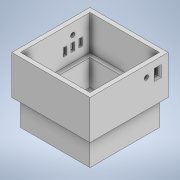
# Autodesk Inventor part: BlackBoxBottomFall2019
Saved by Autodesk Inventor 2020 (Build 240168000, 168)
## iProperties
Created: 2019-08-26
Part Number: BlackBoxBottomFall2019
Material: Generic
Document SubType Name: Modeling
Designer: hwatsky
Density: 1 g/cm^3
Appearance: Default
Author: hwatsky
Autodesk Inventor part; units mm, degrees
ref_plane "YZ Plane" through (0, 0, 0) normal (1, 0, 0) x (0, 1, 0)
ref_plane "XZ Plane" through (0, 0, 0) normal (0, 1, 0) x (-1, 0, 0)
ref_plane "XY Plane" through (0, 0, 0) normal (0, 0, 1) x (1, 0, 0)
sketch "Sketch1" plane through (0, 0, 0) normal (0, 1, 0) x (-1, 0, 0)
  line L0 (0, 0) -> (80, 0)
  line L1 (80, 0) -> (80, -80)
  line L2 (80, -80) -> (0, -80)
  line L3 (0, -80) -> (0, 0)
  dimension "d0" = 80
  dimension "d1" = 80
  constraints: 8 end point, 2 parallel, 1 horizontal, 1 perpendicular
  measures "d0" distance of L0.end L1.end
  measures "d1" distance of L1.end L2.end
extrude "Extrusion1" add sketch "Sketch1" along normal blind 30
sketch "Sketch2" plane through (0, 30, 0) normal (0, 1, 0) x (1, 0, 0)
  line L0 (-85, -5) -> (5, -5)
  line L1 (5, -5) -> (5, 85)
  line L2 (5, 85) -> (-85, 85)
  line L3 (-85, 85) -> (-85, -5)
  line L4 (-80, 80) -> (-80, 0) projected
  line L5 (0, 80) -> (-80, 80) projected
  line L6 (-80, 0) -> (0, 0) projected
  line L7 (0, 0) -> (0, 80) projected
  dimension "d4" = 5
  dimension "d5" = 5
  dimension "d6" = 5
  dimension "d7" = 5
  constraints: 8 end point, 2 parallel, 1 horizontal, 1 perpendicular
  measures "d4" distance between parallel lines of L4 L3
  measures "d5" distance between parallel lines of L2 L5
  measures "d6" distance between parallel lines of L6 L0
  measures "d7" distance between parallel lines of L1 L7
extrude "Extrusion2" add sketch "Sketch2" along normal blind 45 contours L3 L2 L1 L0 | L5 L7 L6 L4
sketch "Sketch3" plane through (0, 75, 0) normal (0, 1, 0) x (1, 0, 0)
  line L0 (0, 0) -> (-80, 0)
  line L1 (-80, 0) -> (-80, 80)
  line L2 (-80, 80) -> (0, 80)
  line L3 (0, 80) -> (0, 0)
  line L4 (-85, 85) -> (-85, -5) projected
  line L5 (5, 85) -> (-85, 85) projected
  dimension "d10" = 5
  dimension "d11" = 5
  constraints: 8 end point, 2 parallel, 1 horizontal, 1 perpendicular
  measures "d10" distance between parallel lines of L4 L1
  measures "d11" distance between parallel lines of L5 L2
extrude "Extrusion3" cut sketch "Sketch3" against normal blind 40
sketch "Sketch4" plane through (0, 35, 0) normal (0, 1, 0) x (1, 0, 0)
  line L0 (-75, 5) -> (-5, 5)
  line L1 (-5, 5) -> (-5, 75)
  line L2 (-5, 75) -> (-75, 75)
  line L3 (-75, 75) -> (-75, 5)
  line L4 (-80, 80) -> (0, 80) projected
  line L5 (0, 80) -> (0, 0) projected
  line L6 (0, 0) -> (-80, 0) projected
  line L7 (-80, 0) -> (-80, 80) projected
  dimension "d14" = 5
  dimension "d15" = 5
  dimension "d16" = 5
  dimension "d17" = 5
  constraints: 8 end point, 2 parallel, 1 horizontal, 1 perpendicular
  measures "d14" distance between parallel lines of L4 L2
  measures "d15" distance between parallel lines of L5 L1
  measures "d16" distance between parallel lines of L6 L0
  measures "d17" distance between parallel lines of L7 L3
extrude "Extrusion4" cut sketch "Sketch4" against normal blind 30 contours L3 L2 L1 L0
sketch "Sketch5" plane through (5, 30, 5) normal (1, 0, 0) x (0, 0, -1)
  circle A0 centre (65, 32.5) radius 2.5
  line L0 (0, 45) -> (90, 45) projected
  line L1 (90, 0) -> (90, 45) projected
  point P0 (5, -30)
  dimension "d20" = 5
  dimension "d21" = 12.5
  dimension "d22" = 25
  constraints: 1 centre point
  measures "d20" diameter of A0
  measures "d21" distance from line of A0.centre L0
  measures "d22" distance from line of L1 A0.centre
extrude "Extrusion5" cut sketch "Sketch5" against normal through all
sketch "Sketch6" plane through (5, 30, 5) normal (1, 0, 0) x (0, 0, -1)
  line L0 (76, 35) -> (80, 35)
  line L1 (80, 35) -> (80, 26)
  line L2 (80, 26) -> (76, 26)
  line L3 (76, 26) -> (76, 35)
  line L4 (90, 0) -> (90, 45) projected
  line L5 (0, 45) -> (90, 45) projected
  point P0 (5, -30)
  dimension "d25" = 10
  dimension "d26" = 4
  dimension "d27" = 9
  dimension "d28" = 10
  constraints: 8 end point, 2 parallel, 1 horizontal, 1 perpendicular
  measures "d25" distance between parallel lines of L4 L1
  measures "d26" distance of L1.end L2.end
  measures "d27" distance of L0.end L1.end
  measures "d28" distance between parallel lines of L0 L5
extrude "Extrusion6" cut sketch "Sketch6" against normal blind 10
chamfer "Chamfer1" distance 2 angle 45 4 edges at (5, 60.5, -71) (5, 65, -73) (5, 60.5, -75) (5, 56, -73)
sketch "Sketch8" plane through (-85, 30, -85) normal (-1, 0, 0) x (0, 0, 1)
  line L0 (23, 25) -> (27, 25)
  line L1 (27, 25) -> (27, 16)
  line L2 (27, 16) -> (23, 16)
  line L3 (23, 16) -> (23, 25)
  line L4 (14, 25) -> (18, 25)
  line L5 (18, 25) -> (18, 16)
  line L6 (18, 16) -> (14, 16)
  line L7 (14, 16) -> (14, 25)
  line L8 (32, 25) -> (36, 25)
  line L9 (36, 25) -> (36, 16)
  line L10 (36, 16) -> (32, 16)
  line L11 (32, 16) -> (32, 25)
  line L12 (0, 45) -> (90, 45) projected
  line L13 (0, 0) -> (0, 45) projected
  point P0 (85, -30)
  dimension "d39" = 4
  dimension "d40" = 9
  dimension "d41" = 4
  dimension "d42" = 4
  dimension "d43" = 20
  dimension "d44" = 23
  dimension "d45" = 5
  dimension "d46" = 5
  constraints: 24 end point, 6 parallel, 4 point on line, 3 horizontal, 3 perpendicular
  measures "d39" distance of L5.end L6.end
  measures "d40" distance of L6.end L4.start
  measures "d41" distance of L1.end L2.end
  measures "d42" distance of L9.end L10.end
  measures "d43" distance between parallel lines of L12 L4
  measures "d44" distance between parallel lines of L13 L3
  measures "d45" distance between parallel lines of L3 L5
  measures "d46" distance between parallel lines of L11 L1
extrude "Extrusion7" cut sketch "Sketch8" against normal blind 10
chamfer "Chamfer2" distance 2 angle 45 12 edges at (-85, 55, -69) (-85, 50.5, -71) (-85, 50.5, -67) (-85, 46, -69) (-85, 50.5, -62) (-85, 55, -60) (-85, 50.5, -58) (-85, 46, -60) (-85, 50.5, -53) (-85, 55, -51) (-85, 50.5, -49) (-85, 46, -51)
body "Solid1"
